Bottom Plate VPD CNC_v8 (Autodesk Fusion 360 design; units mm, degrees)
Autodesk Fusion 360 part; units mm, degrees
note: some values were not read from the file. Chosen so that the rebuilt part matches the saved one: which face or edge a step refers to.
sketch "Sketch1" plane through (0, 0, 0) normal (0, 1, 0) x (1, 0, 0)
  line L0 (110, 110) -> (-110, 110)
  line L1 (-110, 110) -> (-110, -110)
  line L2 (-110, -110) -> (110, -110)
  line L3 (110, -110) -> (110, 110)
  line L4 (110, 110) -> (-110, -110) construction
  line L5 (-110, 110) -> (110, -110) construction
  circle A0 centre (0, 0) radius 82.5
  circle A1 centre (-85.5, -85.5) radius 15
  circle A2 centre (85.5, -85.5) radius 15
  circle A3 centre (85.5, 85.5) radius 15
  circle A4 centre (-85.5, 85.5) radius 15
  line L6 (0, -110) -> (0, 0) construction
  line L7 (-20, -110) -> (-20, -80.0391)
  line L8 (20, -110) -> (20, -80.0391)
  point P0 (-85.5, -85.5)
  point P1 (85.5, -85.5)
  point P2 (85.5, 85.5)
  point P3 (-85.5, 85.5)
  dimension "d1" = 220
  dimension "d2" = 220
  dimension "d3" = 24.5
  dimension "d4" = 24.5
  dimension "d6" = 360
  dimension "d11" = 165
  dimension "d13" = 30
  dimension "d15" = 360
  dimension "d41" = 20
  constraint horizontal L0
  constraint perpendicular L0 L1
  constraint parallel L0 L2
  constraint parallel L1 L3
  constraint coincident L4 A0.centre
  constraint coincident L5 A0.centre
  constraint coincident A0.centre L6.end
  constraint coincident L4 P0
  constraint coincident P0 A1.centre
  constraint midpoint L2 L6.start
  constraint coincident L2 L7.start
  constraint coincident A0 L7.end
  constraint perpendicular L2 L7
  constraint symmetric L6 L7.start L8.start
  constraint symmetric L6 L7.end L8.end
  measures "d1" distance of L0.end L1.end
  measures "d2" distance of L1.end L2.end
  measures "d3" distance of L1 P0
  measures "d4" distance of L2 P0
  measures "d11" diameter of A0
  measures "d13" diameter of A1
  measures "d41" distance of L6 L7
extrude "Extrude1" add sketch "Sketch1" along normal blind 2 contours L0 L1 L2 L3 A0 L7 L8 | L2 A0 L7 L8 | A0 | A1 | A2 | A3 | A4
sketch "Sketch2" plane through (0, 2, 0) normal (0, 1, 0) x (-1, 0, 0)
  line L0 (-110, 110) -> (-110, -110)
  line L1 (-110, -110) -> (110, -110)
  line L2 (110, -110) -> (110, 110)
  line L3 (110, 110) -> (-110, 110)
  point P0 (85.5, 85.5)
extrude "Extrude2" add sketch "Sketch1" along normal blind 13 from surface at 2 contours L0 L1 L2 L3 A0 L7 L8 | A2 | A3 | A4
sketch "Sketch3" plane through (0, 15, 0) normal (0, 1, 0) x (-1, 0, 0)
  line L0 (110, 110) -> (20, 110)
  line L1 (-110, 110) -> (-110, -110)
  line L2 (-110, -110) -> (110, -110)
  line L3 (110, -110) -> (110, 110)
  circle A0 centre (85.5, 85.5) radius 15
  line L4 (20, 110) -> (20, 80.0391)
  arc A1 (-20, 80.0391) -> (20, 80.0391) centre (0, 0) ccw
  line L5 (-20, 80.0391) -> (-20, 110)
  line L6 (-20, 110) -> (-110, 110)
  point P0 (85.5, -85.5)
  point P1 (-85.5, -85.5)
  point P2 (85.5, 85.5)
  point P3 (-85.5, 85.5)
hole "Hole3" at (-85.5, 15, -85.5) at (85.5, 15, -85.5) at (-85.5, 15, 85.5) at (85.5, 15, 85.5) direction (0, -1, 0) diameter 4.5 depth 15 tip angle 180
hole "Hole5" at (-85.5, 15, -85.5) at (-85.5, 15, 85.5) at (85.5, 15, 85.5) at (85.5, 15, -85.5) direction (0, -1, 0) diameter 9.4 depth 13 tip angle 118
pattern_circular "C-Pattern1" count 2 over 90 about axis through (0, 1.75, 0) along (0, 1, 0) of 2 faces at (-18.0717, 2, -0.8052) (-70.5745, 6.3333, 86.9935)
equation "overall_height = 15 mm"
equation "cutout_depth = 13 mm"
equation "wafer_slot_diameter = 165 mm"
equation "cuevette_slot_diam = 30 mm"
equation "d11 = wafer_slot_diameter"
equation "screw_plate_thickness = 2 mm"
equation "d13 = cuevette_slot_diam"
equation "d16 = screw_plate_thickness"
equation "d18 = overall_height - screw_plate_thickness"
equation "d20 = screw_plate_thickness"
equation "d42 = overall_height - screw_plate_thickness"
